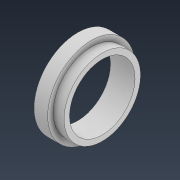
# Autodesk Inventor part: Mocowanie uszczelki tyl
Saved by Autodesk Inventor 2022 (Build 260153000, 153)
## iProperties
Created: 2023-04-12
Part Number: Mocowanie uszczelki tyl
Material: Generic
Document SubType Name: Modeling
Designer: wikto
Density: 1 g/cm^3
Appearance: Default
Author: wikto
Autodesk Inventor part; units mm, degrees
ref_plane "YZ Plane" through (0, 0, 0) normal (1, 0, 0) x (0, 1, 0)
ref_plane "XZ Plane" through (0, 0, 0) normal (0, 1, 0) x (-1, 0, 0)
ref_plane "XY Plane" through (0, 0, 0) normal (0, 0, 1) x (1, 0, 0)
sketch "Sketch1" plane through (0, 0, 0) normal (0, 0, 1) x (1, 0, 0)
  line L0 (0, 0) -> (100, 0)
  line L1 (0, 12) -> (9, 12)
  line L2 (9, 12) -> (9, 14)
  line L3 (9, 14) -> (5, 14)
  line L4 (5, 14) -> (5, 16)
  line L5 (5, 16) -> (0, 16)
  line L6 (0, 16) -> (0, 12)
  dimension "d0" = 100
  dimension "d1" = 32
  dimension "d2" = 9
  dimension "d3" = 4
  dimension "d4" = 28
  dimension "d5" = 24
  constraints: 14 end point, 5 perpendicular, 2 horizontal, 1 vertical alignment
  measures "d0" distance of L0.start L0.end
  measures "d1" diameter of L5 L0
  measures "d2" distance between parallel lines of L6 L2
  measures "d3" distance between parallel lines of L4 L2
  measures "d4" diameter of L3 L0
  measures "d5" diameter of L1 L0
revolve "Revolution1" add sketch "Sketch1" angle 360 about axis through (0, 0, 0) along (1, 0, 0)
body "Solid1"
